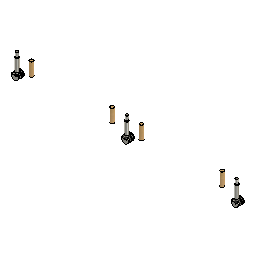
Minifix D15 Set (Autodesk Fusion 360 design; units mm, degrees)
description: Connecting Bolt
part number: L34
description: Dowel
part number: 8x30
description: Minifix CAM
part number: D15
description: Minifix Cap
part number: Minifix Cap D15
Autodesk Fusion 360 part; units mm, degrees
sketch "Main Area" plane through (0, 0, 0) normal (0, 0, 1) x (1, 0, 0)
  line L0 (300, 9) -> (-300, 9)
  line L1 (-300, 9) -> (-300, -9)
  line L2 (-300, -9) -> (300, -9)
  line L3 (300, -9) -> (300, 9)
  line L4 (300, 9) -> (-300, -9) construction
  line L5 (-300, 9) -> (300, -9) construction
  dimension "d3" = 600
  dimension "d4" = 18
  constraint horizontal L0
  constraint perpendicular L0 L1
  constraint parallel L0 L2
  constraint parallel L1 L3
  constraint coincident L4 origin
  constraint coincident L5 origin
  measures "d3" distance of L1.end L2.end
  measures "d4" distance of L0.end L1.end
sketch "Minfix Calc" plane through (0, 0, 0) normal (0, 0, 1) x (1, 0, 0)
  line L0 (0, 40) -> (0, -50)
  circle A0 centre (240, 1) radius 0.5
  line L1 (300, -9) -> (300, 9)
  line L2 (300, 9) -> (-300, 9)
  circle A1 centre (-240, 1) radius 0.5
  line L3 (-300, 9) -> (-300, -9)
  dimension "d7" = 1
  dimension "d8" = 60
  dimension "d9" = 8
  dimension "d18" = 1
  dimension "d19" = 8
  dimension "d20" = 60
  constraint vertical L0
  measures "d7" diameter of A0
  measures "d8" distance of A0.centre L1
  measures "d9" distance of A0.centre L2
  measures "d18" diameter of A1
  measures "d19" distance of L2 A1.centre
  measures "d20" distance of A1.centre L3
extrude "Extrude1" add sketch "Minfix Calc" along normal blind 10 contours A0 makes body 1
extrude "Extrude2" add sketch "Minfix Calc" along normal blind 10 separate body contours A1 makes body 2
sketch "Dowel Calc" plane through (0, 0, 0) normal (0, 0, 1) x (1, 0, 0)
  circle A0 centre (208, 1) radius 0.5
  circle A1 centre (240, 1) radius 0.5
  circle A2 centre (-208, 1) radius 0.5
  circle A3 centre (-240, 1) radius 0.5
  line L0 (-300, 9) -> (-300, -9)
  line L1 (300, -9) -> (300, 9)
  dimension "d23" = 1
  dimension "d25" = 1
  dimension "d55" = 92
  dimension "d56" = 92
  constraint horizontal A0.centre A1.centre
  constraint horizontal A2.centre A3.centre
  measures "d23" diameter of A0
  measures "d25" diameter of A2
  measures "d55" distance of A2.centre L0
  measures "d56" distance of A0.centre L1
extrude "Extrude3" add sketch "Dowel Calc" along normal blind 10 separate body contours A0 makes body 3
extrude "Extrude4" add sketch "Dowel Calc" along normal blind 10 separate body contours A2 makes body 4
pattern_linear "R-Pattern1" count 2 spacing 240 along (-1, 0, 0) of bodies 1 makes body 5
pattern_linear "R-Pattern3" count 2 spacing 240 along (-1, 0, 0) of bodies 3 makes body 6
pattern_linear "R-Pattern4" count 2 spacing 240 along (1, 0, 0) of bodies 4 makes body 7
sketch "Sketch6" plane through (0, 0, 0) normal (0, 0, 1) x (1, 0, 0)
  circle A0 centre (240, 1) radius 0.5
  circle A1 centre (240, 1) radius 2.5
  dimension "d57" = 5
  constraint concentric A0 A1
  measures "d57" diameter of A1
extrude "Extrude1'" add sketch "Sketch6" along normal blind 1.6 separate body contours A0 | A1 makes body 8 in component "Minifix Right"
sketch "Sketch1" plane through (0, 0, 1.6) normal (0, 0, 1) x (-1, 0, 0) in component "Minifix Right"
  circle A0 centre (-240, -1) radius 2.5
  circle A1 centre (-240, -1) radius 3
  dimension "d64" = 6
  constraint concentric A0 A1
  measures "d64" diameter of A1
extrude "Extrude2'" add sketch "Sketch1" along normal blind 9.4 contours A0 | A1 bodies 8 in component "Minifix Right"
chamfer "Chamfer1" distance 0.5 angle 45 1 edges at (242.797, 2.0848, 11) on bodies 8 in component "Minifix Right"
thread "Thread1" "ISO Metric profile 6.0 M6x1 6g" major diameter 5.884 minor diameter 4.7435 pitch 1 angle 60 resizes the face on face at (239.1875, -1.8879, 7.5333) on bodies 8 in component "Minifix Right"
sketch "Sketch2" plane through (0, 0, 0) normal (0, 0, -1) x (1, 0, 0) in component "Minifix Right"
  circle A0 centre (240, -1) radius 2.5
  circle A1 centre (240, -1) radius 2
  dimension "d68" = 4
  constraint concentric A0 A1
  measures "d68" diameter of A1
extrude "Extrude3'" add sketch "Sketch2" along normal blind 34 contours A1 bodies 8 in component "Minifix Right"
sketch "Sketch3" plane through (0, 0, -34) normal (0, 0, -1) x (1, 0, 0) in component "Minifix Right"
  circle A0 centre (240, -1) radius 2
  circle A1 centre (240, -1) radius 3.25
  line L0 (243.25, -1) -> (236.75, -1)
  dimension "d72" = 6.5
  constraint concentric A0 A1
  constraint horizontal L0
  constraint coincident A1 L0.start
  constraint coincident A1 L0.end
  constraint coincident A0.centre L0
  measures "d72" diameter of A1
revolve "Revolve1" add sketch "Sketch3" angle 180 about axis through (243.25, 1, -34) along (1, 0, 0) contours A0 A1 L0 picked at (237.1788, -1.1615) bodies 8 in component "Minifix Right"
sketch "Sketch4" plane through (0, 0, 0) normal (0, 0, -1) x (1, 0, 0) in component "Minifix Right"
  circle A0 centre (240, -1) radius 2
  circle A1 centre (240, -1) radius 2.5
  circle A2 centre (240, -1) radius 4
  dimension "d74" = 8
  constraint concentric A0 A2
  measures "d74" diameter of A2
ref_plane "WorkPlane1" through (240, 1, -26) normal (0, 0, -1) x (1, 0, 0) in component "Minifix Right"
extrude "Extrude4'" add sketch "Sketch4" along normal up to surface (26 mm away) contours A1 | A2 bodies 8 in component "Minifix Right"
sketch "Sketch5" plane through (0, 0, -34) normal (0, 0, -1) x (1, 0, 0) in component "Minifix Right"
  circle A0 centre (240, -1) radius 3.25
  line L0 (236.5, -0.5) -> (243.5, -0.5)
  line L1 (243.5, -0.5) -> (243.5, -1.5)
  line L2 (243.5, -1.5) -> (236.5, -1.5)
  line L3 (236.5, -1.5) -> (236.5, -0.5)
  line L4 (236.5, -0.5) -> (243.5, -1.5) construction
  line L5 (243.5, -0.5) -> (236.5, -1.5) construction
  line L6 (239.5, 2.5) -> (240.5, 2.5)
  line L7 (240.5, 2.5) -> (240.5, -4.5)
  line L8 (240.5, -4.5) -> (239.5, -4.5)
  line L9 (239.5, -4.5) -> (239.5, 2.5)
  line L10 (239.5, 2.5) -> (240.5, -4.5) construction
  line L11 (240.5, 2.5) -> (239.5, -4.5) construction
  point P0 (240, -1)
  point P1 (240, -1)
  dimension "d78" = 1
  dimension "d79" = 1
  dimension "d82" = 3.5
  dimension "d83" = 3.5
  constraint horizontal L0
  constraint perpendicular L0 L1
  constraint parallel L0 L2
  constraint parallel L1 L3
  constraint coincident L4 P1
  constraint coincident L5 P1
  constraint coincident P0 A0.centre
  constraint horizontal L6
  constraint perpendicular L6 L7
  constraint parallel L6 L8
  constraint parallel L7 L9
  constraint coincident L10 P1
  constraint coincident L11 P1
  constraint coincident P1 P0
  measures "d78" distance of L0.end L1.end
  measures "d79" distance of L7.end L8.end
  measures "d82" distance of L3 P1
  measures "d83" distance of P1 L8
extrude "Extrude5" cut sketch "Sketch5" against normal blind 1.5 draft -10 contours A0 L0 L2 L7 | A0 L0 L1 L2 | A0 L0 L7 L9 | A0 L6 L7 L9 | L0 L2 L7 L9 | A0 L7 L8 L9 | A0 L2 L7 L9 | A0 L0 L2 L9 | A0 L0 L2 L3 bodies 8 in component "Minifix Right"
sketch "Sketch6 (2)" plane through (0, 0, 0) normal (0, 0, 1) x (-1, 0, 0) in component "Minifix Right"
  circle A0 centre (-240, -1) radius 4
  circle A1 centre (-240, -1) radius 2.5
  circle A2 centre (-240, -1) radius 4
  dimension "d84" = 8
  constraint concentric A0 A2
  measures "d84" diameter of A2
extrude "Extrude6" add sketch "Sketch6 (2)" against normal blind 34 separate body contours A0 A2 | A1 makes body 9 in component "Minifix Right"
sketch "Sketch7" plane through (0, 0, 0) normal (0, 0, 1) x (-1, 0, 0) in component "Minifix Right"
  circle A0 centre (-240, -1) radius 4
  circle A1 centre (-240, -1) radius 2.5
  dimension "d87" = 5
  constraint concentric A0 A1
  measures "d87" diameter of A1
extrude "Extrude7" add sketch "Sketch7" along normal blind 13 contours A1 bodies 9 in component "Minifix Right"
pattern_linear "00000000-0000-0000-0000-000000000000" [suppressed]
sketch "Sketch7 (2)" plane through (0, 0, 0) normal (0, 0, 1) x (1, 0, 0)
  circle A0 centre (-240, 1) radius 0.5
  circle A1 centre (-240, 1) radius 2.5
  dimension "d94" = 5
  constraint concentric A0 A1
  measures "d94" diameter of A1
extrude "Extrude1''" add sketch "Sketch7 (2)" along normal blind 1.6 separate body contours A0 | A1 makes body 10 in component "Minifix left"
sketch "Sketch1 (2)" plane through (0, 0, 1.6) normal (0, 0, 1) x (-1, 0, 0) in component "Minifix left"
  circle A0 centre (240, -1) radius 2.5
  circle A1 centre (240, -1) radius 3
  dimension "d101" = 6
  constraint concentric A0 A1
  measures "d101" diameter of A1
extrude "Extrude2''" add sketch "Sketch1 (2)" along normal blind 9.4 contours A0 | A1 bodies 10 in component "Minifix left"
chamfer "Chamfer1'" distance 0.5 angle 45 1 edges at (-237.203, 2.0848, 11) on bodies 10 in component "Minifix left"
thread "Thread1'" "ISO Metric profile 6.0 M6x1 6g" major diameter 5.884 minor diameter 4.7435 pitch 1 angle 60 resizes the face on face at (-240.9555, -1.8438, 7.5333) on bodies 10 in component "Minifix left"
sketch "Sketch2 (2)" plane through (0, 0, 0) normal (0, 0, -1) x (1, 0, 0) in component "Minifix left"
  circle A0 centre (-240, -1) radius 2.5
  circle A1 centre (-240, -1) radius 2
  dimension "d105" = 4
  constraint concentric A0 A1
  measures "d105" diameter of A1
extrude "Extrude3''" add sketch "Sketch2 (2)" along normal blind 34 contours A1 bodies 10 in component "Minifix left"
sketch "Sketch5 (2)" plane through (0, 0, -34) normal (0, 0, -1) x (1, 0, 0) in component "Minifix left"
  circle A0 centre (-240, -1) radius 2
  line L0 (-236.75, -1) -> (-243.25, -1)
  arc A1 (-243.25, -1) -> (-236.75, -1) centre (-240, -1) ccw
  dimension "d110" = 6.5
  constraint concentric A0 A1
  constraint horizontal L0
  constraint coincident L0 A1.end
  constraint coincident L0 A1.start
  constraint coincident L0.start A1.end
  constraint coincident L0.end A1.start
  constraint coincident A0.centre L0
  measures "d110" diameter of A1
revolve "Revolve1'" add sketch "Sketch5 (2)" angle 180 about axis through (-236.75, 1, -34) along (1, 0, 0) contours A0 L0 A1 | A0 L0 picked at (-239.6702, -2.1926) bodies 10 in component "Minifix left"
sketch "Sketch6 (3)" plane through (0, 0, 0) normal (0, 0, -1) x (1, 0, 0) in component "Minifix left"
  circle A0 centre (-240, -1) radius 2
  circle A1 centre (-240, -1) radius 2.5
  circle A2 centre (-240, -1) radius 4
  dimension "d112" = 8
  constraint concentric A0 A2
  measures "d112" diameter of A2
extrude "Extrude4''" add sketch "Sketch6 (3)" along normal up to surface (26 mm away) contours A1 | A2 bodies 10 in component "Minifix left"
sketch "Sketch7 (3)" plane through (0, 0, -34) normal (0, 0, -1) x (1, 0, 0) in component "Minifix left"
  circle A0 centre (-240, -1) radius 3.25
  line L0 (-243.5, -0.5) -> (-236.5, -0.5)
  line L1 (-236.5, -0.5) -> (-236.5, -1.5)
  line L2 (-236.5, -1.5) -> (-243.5, -1.5)
  line L3 (-243.5, -1.5) -> (-243.5, -0.5)
  line L4 (-243.5, -0.5) -> (-236.5, -1.5) construction
  line L5 (-236.5, -0.5) -> (-243.5, -1.5) construction
  line L6 (-240.5, 2.5) -> (-239.5, 2.5)
  line L7 (-239.5, 2.5) -> (-239.5, -4.5)
  line L8 (-239.5, -4.5) -> (-240.5, -4.5)
  line L9 (-240.5, -4.5) -> (-240.5, 2.5)
  line L10 (-240.5, 2.5) -> (-239.5, -4.5) construction
  line L11 (-239.5, 2.5) -> (-240.5, -4.5) construction
  point P0 (-240, -1)
  point P1 (-240, -1)
  dimension "d115" = 1
  dimension "d116" = 1
  dimension "d119" = 3.5
  dimension "d120" = 3.5
  constraint horizontal L0
  constraint perpendicular L0 L1
  constraint parallel L0 L2
  constraint parallel L1 L3
  constraint coincident L4 P1
  constraint coincident L5 P1
  constraint coincident P0 A0.centre
  constraint horizontal L6
  constraint perpendicular L6 L7
  constraint parallel L6 L8
  constraint parallel L7 L9
  constraint coincident L10 P1
  constraint coincident L11 P1
  constraint coincident P1 P0
  measures "d115" distance of L0.end L1.end
  measures "d116" distance of L7.end L8.end
  measures "d119" distance of L3 P1
  measures "d120" distance of L8 P1
extrude "Extrude5'" cut sketch "Sketch7 (3)" against normal blind 1.5 draft -5 contours A0 L0 L2 L7 | A0 L0 L1 L2 | A0 L0 L7 L9 | A0 L6 L7 L9 | L0 L2 L7 L9 | A0 L7 L8 L9 | A0 L2 L7 L9 | A0 L0 L2 L9 | A0 L0 L2 L3 bodies 10 in component "Minifix left"
sketch "Sketch8" plane through (0, 0, 0) normal (0, 0, 1) x (-1, 0, 0) in component "Minifix left"
  circle A0 centre (240, -1) radius 4
  circle A1 centre (240, -1) radius 2.5
  circle A2 centre (240, -1) radius 4
  dimension "d121" = 8
  constraint concentric A0 A2
  measures "d121" diameter of A2
extrude "Extrude6'" add sketch "Sketch8" against normal blind 34 separate body contours A0 A2 | A1 makes body 11 in component "Minifix left"
sketch "Sketch9" plane through (0, 0, 0) normal (0, 0, 1) x (-1, 0, 0) in component "Minifix left"
  circle A0 centre (240, -1) radius 4
  circle A1 centre (240, -1) radius 2.5
  dimension "d124" = 5
  constraint concentric A0 A1
  measures "d124" diameter of A1
extrude "Extrude7'" add sketch "Sketch9" along normal blind 13 contours A1 bodies 11 in component "Minifix left"
sketch "Sketch8 (2)" plane through (0, 0, 0) normal (0, 0, 1) x (1, 0, 0)
  circle A0 centre (208, 1) radius 0.5
  circle A1 centre (208, 1) radius 4
  dimension "d132" = 8
  constraint concentric A0 A1
  measures "d132" diameter of A1
extrude "Extrude1'''" add sketch "Sketch8 (2)" along normal blind 10 and the other way blind 20 separate body contours A0 | A1 makes body 12 in component "Dowel Right"
chamfer "Chamfer1''" distance 0.5 angle 45 2 edges at (204.2707, 2.4465, -20) (204.2707, -0.4465, 10) on bodies 12 in component "Dowel Right"
extrude "Extrude2'''" add sketch "Sketch8 (2)" along normal blind -30 and the other way blind -12 separate body contours A0 | A1 makes body 13 in component "Dowel Right"
pattern_linear "00000000-0000-0000-0000-000000000000'" [suppressed]
sketch "Sketch9 (2)" plane through (0, 0, 10) normal (0, 0, 1) x (-1, 0, 0)
  circle A0 centre (208, -1) radius 0.5
  circle A1 centre (208, -1) radius 0.5
  circle A2 centre (208, -1) radius 4
  dimension "d150" = 8
  constraint concentric A1 A2
  measures "d150" diameter of A2
extrude "Extrude1''''" add sketch "Sketch9 (2)" along normal blind 10 and the other way blind 20 separate body contours A0 A1 | A2 makes body 14 in component "Dowel Left"
chamfer "Chamfer1'''" distance 0.5 angle 45 2 edges at (-204.2707, -0.4465, -10) (-204.2707, 2.4465, 20) on bodies 14 in component "Dowel Left"
extrude "Extrude2''''" add sketch "Sketch9 (2)" along normal blind 2 and the other way blind 40 separate body contours A0 A1 | A2 sketch seen with x (1, 0, 0) y (0, 1, 0) z (0, 0, 1) at (0, 0, 10) makes body 15 in component "Dowel Left"
pattern_linear "00000000-0000-0000-0000-000000000000''" [suppressed]
ref_plane "WorkPlane1" through (240, 1, -13) normal (0, 1, 0) x (0, 0, -1)
ref_plane "WorkPlane2" through (240, -3.5, -13) normal (0, 1, 0) x (0, 0, -1)
sketch "Sketch11" plane through (240, -3.5, -13) normal (0, 1, 0) x (1, 0, 0)
  line L0 (-0.5, 21) -> (0.5, 21) construction
  circle A0 centre (0, 21) radius 7.5
  point P0 (-0.5, 21)
  point P1 (0.5, 21)
  point P2 (0, 21)
  dimension "d170" = 15
  constraint coincident P0 L0.start
  constraint coincident P1 L0.end
  constraint midpoint L0 P2
  constraint coincident P2 A0.centre
  measures "d170" diameter of A0
extrude "Extrude1'''''" add sketch "Sketch11" along normal blind 12.5 separate body makes body 16 in component "Minifix CAM Right"
sketch "Sketch1 (3)" plane through (0, 9, 0) normal (0, 1, 0) x (-1, 0, 0) in component "Minifix CAM Right"
  circle A0 centre (-240, -34) radius 7.5
  circle A1 centre (-240, -34) radius 5.5 construction
  line L0 (-245.4486, -33.25) -> (-234.5514, -33.25)
  line L1 (-234.5514, -33.25) -> (-234.5514, -34.75)
  line L2 (-234.5514, -34.75) -> (-245.4486, -34.75)
  line L3 (-245.4486, -34.75) -> (-245.4486, -33.25)
  line L4 (-245.4486, -33.25) -> (-234.5514, -34.75) construction
  line L5 (-234.5514, -33.25) -> (-245.4486, -34.75) construction
  line L6 (-240.75, -39.4486) -> (-239.25, -39.4486)
  line L7 (-239.25, -39.4486) -> (-239.25, -28.5514)
  line L8 (-239.25, -28.5514) -> (-240.75, -28.5514)
  line L9 (-240.75, -28.5514) -> (-240.75, -39.4486)
  line L10 (-240.75, -39.4486) -> (-239.25, -28.5514) construction
  line L11 (-239.25, -39.4486) -> (-240.75, -28.5514) construction
  point P0 (-240, -34)
  point P1 (-240, -34)
  dimension "d174" = -2
  dimension "d175" = 1.5
  dimension "d176" = 1.5
  constraint horizontal L0
  constraint perpendicular L0 L1
  constraint parallel L0 L2
  constraint parallel L1 L3
  constraint coincident L4 P1
  constraint coincident L5 P1
  constraint coincident P0 A0.centre
  constraint horizontal L6
  constraint perpendicular L6 L7
  constraint parallel L6 L8
  constraint parallel L7 L9
  constraint coincident L10 P1
  constraint coincident L11 P1
  constraint coincident P1 P0
  constraint coincident A1 L6.end
  constraint coincident A1 L2.end
  measures "d175" distance of L0.end L1.end
  measures "d176" distance of L7.end L8.end
extrude "Extrude2'''''" cut sketch "Sketch1 (3)" against normal blind 2 draft -4 contours L0 L2 L3 L9 | L0 L7 L8 L9 | L0 L2 L7 L9 | L0 L1 L2 L7 | L2 L6 L7 L9 bodies 16 in component "Minifix CAM Right"
ref_plane "WorkPlane1" through (240, 3.5, -34) normal (0, 0, 1) x (0, 1, 0) in component "Minifix CAM Right"
sketch "Sketch2 (3)" plane through (240, 1.5, -34) normal (0, 0, 1) x (1, 0, 0) in component "Minifix CAM Right"
  circle A0 centre (0, -0.5) radius 2.25
  line L0 (7.5, 7.5) -> (-7.5, 7.5)
  line L1 (0, 1.75) -> (7.5, 1.75)
  line L2 (0, -2.75) -> (7.5, -2.75)
  line L3 (7.5, 7.5) -> (-7.5, 7.5)
  line L4 (7.5, -5) -> (-7.5, -5)
  line L5 (7.5, 7.5) -> (7.5, -5)
  line L6 (7.5, -5) -> (-7.5, -5)
  point P0 (0, -5)
  dimension "d181" = 4.5
  dimension "d182" = 8
  constraint horizontal L1
  constraint parallel L1 L2
  constraint tangent A0 L1
  constraint coincident A0 L1.start
  constraint coincident A0 L2.start
  constraint coincident L0.start L3.start
  constraint coincident L4.start L5.end
  constraint coincident L1.end L5
  constraint coincident L2.end L5
  constraint tangent A0 L2
  constraint midpoint L4 P0
  constraint vertical A0.centre P0
  measures "d181" diameter of A0
  measures "d182" distance of A0.centre L0
extrude "Extrude3'''" cut sketch "Sketch2 (3)" along normal mid plane 22 bodies 16 in component "Minifix CAM Right"
sketch "Sketch3 (2)" plane through (0, -3.5, 0) normal (0, -1, 0) x (1, 0, 0) in component "Minifix CAM Right"
  line L0 (245, -33) -> (235, -33)
  line L1 (235, -33) -> (235, -26.5)
  line L2 (235, -26.5) -> (245, -26.5)
  line L3 (245, -26.5) -> (245, -33)
  line L4 (245, -33) -> (235, -26.5) construction
  line L5 (235, -33) -> (245, -26.5) construction
  circle A0 centre (240, -34) radius 7.5
  circle A1 centre (240, -34) radius 7.5
  point P0 (240, -29.75)
  dimension "d186" = 10
  dimension "d274" = 6.5
  constraint horizontal L0
  constraint perpendicular L0 L1
  constraint parallel L0 L2
  constraint parallel L1 L3
  constraint coincident L4 P0
  constraint coincident L5 P0
  constraint tangent L2 A0
  constraint vertical P0 A0.centre
  measures "d186" distance of L1 L3
  measures "d274" distance of L0.end L1.end
extrude "Extrude4'''" cut sketch "Sketch3 (2)" against normal up to surface (6.75 mm away) contours L0 L1 L3 A0 A1 | L2 L3 A0 A1 | L1 L2 A0 A1 picked at (240, -30.8333) bodies 16 in component "Minifix CAM Right"
sketch "Sketch5 (3)" plane through (240, 1.5, -34) normal (0, 0, 1) x (1, 0, 0) in component "Minifix CAM Right"
  line L0 (5, -2.75) -> (5, -5)
  arc A0 (0, 1.75) -> (0, -2.75) centre (0, -0.5) ccw
  circle A1 centre (0, -0.5) radius 3.25
  line L1 (0, 2.75) -> (5, 2.75)
  line L2 (5, 2.75) -> (5, -3.75)
  line L3 (5, -3.75) -> (0, -3.75)
  line L4 (0, -3.75) -> (0, 2.75) construction
  line L5 (7.5, 1.75) -> (-5, 1.75)
  dimension "d191" = 6.5
  constraint concentric A0 A1
  constraint horizontal L1
  constraint vertical L2
  constraint horizontal L3
  constraint vertical L4
  constraint tangent A1 L1
  constraint tangent A1 L3
  constraint collinear L0 L2
  constraint coincident A0.centre L4
  measures "d191" diameter of A1
extrude "Extrude5''" cut sketch "Sketch5 (3)" along normal blind 7.5 and the other way blind 3 contours A1 L1 L2 L5 | A1 L5 | A1 L5 bodies 16 in component "Minifix CAM Right"
move_face "OffsetFaces1" offset -1 1 faces at (235.8849, 3.25, -31.4699) on bodies 16 in component "Minifix CAM Right"
fillet "Fillet1" radius 2 1 edges at (245, 3.75, -37) on bodies 16 in component "Minifix CAM Right"
fillet "Fillet1" radius 2 2 edges at (235, 0.375, -33) (245, -2.375, -33) on bodies 16 in component "Minifix CAM Right"
fillet "Fillet2" radius 1 4 edges at (237.0104, -0.2748, -37) (241.5, 4.25, -37) (244.4142, 4.25, -36.4142) (245, 4.25, -31.7049) on bodies 16 in component "Minifix CAM Right"
fillet "Fillet2" radius 1 3 edges at (238.5, 4.25, -33) (235.5858, 4.25, -32.4142) (235, 4.25, -29.7049) on bodies 16 in component "Minifix CAM Right"
ref_plane "WorkPlane2" through (240, 8, -34) normal (0, 1, 0) x (1, 0, 0) in component "Minifix CAM Right"
ref_plane "WorkPlane3" through (240, 5.25, -30.4688) normal (0, -1, 0) x (1, 0, 0) in component "Minifix CAM Right"
sketch "Sketch6 (4)" plane through (240, 8, -34) normal (0, 1, 0) x (1, 0, 0) in component "Minifix CAM Right"
  line L0 (0.6101, -0.6101) -> (5.3088, -0.6101)
  line L1 (0.6101, -5.3088) -> (0.6101, -0.6101)
  line L2 (-0.6101, -5.3088) -> (0.6101, -5.3088)
  line L3 (-0.6101, -0.6101) -> (-0.6101, -5.3088)
  line L4 (-5.3088, -0.6101) -> (-0.6101, -0.6101)
  line L5 (-0.6101, 0.6101) -> (-5.3088, 0.6101)
  line L6 (-5.3088, 0.6101) -> (-5.3088, -0.6101)
  line L7 (-0.6101, 5.3088) -> (-0.6101, 0.6101)
  line L8 (0.6101, 5.3088) -> (-0.6101, 5.3088)
  line L9 (0.6101, 0.6101) -> (0.6101, 5.3088)
  line L10 (5.3088, 0.6101) -> (0.6101, 0.6101)
  line L11 (5.3088, -0.6101) -> (5.3088, 0.6101)
  arc A0 (5, -5.5902) -> (0, 7.5) centre (0, 0) ccw
  spline S0 degree 3 poles (0, 7.5) (-0.2844, 7.5) (-0.5865, 7.4822) (-1.1404, 7.418) (-1.3922, 7.3725) (-1.7898, 7.2862) (-1.9627, 7.2396) (-2.1928, 7.1733) (-2.25, 7.1545) (-2.25, 7.1545) knots 0.341299 0.341299 0.341299 0.341299 0.426611 0.426611 0.511923 0.511923 0.59726 0.59726 0.682597 0.682597 0.682597 0.682597
  spline S1 degree 3 poles (-4, -6.3443) (-4.1326, -6.2607) (-4.2719, -6.1665) (-4.5277, -5.9812) (-4.6442, -5.8903) (-4.8117, -5.7539) (-4.8804, -5.6952) (-4.9747, -5.613) (-5, -5.5902) (-5, -5.5902) knots 0.161333 0.161333 0.161333 0.161333 0.208345 0.208345 0.255357 0.255357 0.293184 0.293184 0.331011 0.331011 0.331011 0.331011
  spline S2 degree 3 poles (5, -5.5902) (5, -5.5902) (4.9747, -5.613) (4.8804, -5.6952) (4.8117, -5.7539) (4.6442, -5.8903) (4.5277, -5.9812) (4.2719, -6.1665) (4.1326, -6.2607) (4, -6.3443) knots 0 0 0 0 0.037827 0.037827 0.075653 0.075653 0.122665 0.122665 0.169678 0.169678 0.169678 0.169678
  arc A1 (-4, -6.3443) -> (4, -6.3443) centre (0, 0) ccw
  arc A2 (-50.2768, -27.739) -> (-56.5684, 9.8605) centre (0, 0) ccw
  line L12 (-50.2768, -27.739) -> (-49.8166, 6.7466)
  spline S3 degree 3 poles (-49.8166, 6.7466) (-49.8164, 6.7433) (-49.8148, 6.716) (-49.8129, 6.668) (-49.8107, 6.6156) (-49.8082, 6.5341) (-49.8076, 6.4521) (-49.8068, 6.3498) (-49.8085, 6.2191) (-49.8151, 6.0836) (-49.8217, 5.9489) (-49.8338, 5.7996) (-49.849, 5.6667) knots 0.005365 0.005365 0.005365 0.005365 0.037827 0.037827 0.037827 0.075653 0.075653 0.075653 0.122665 0.122665 0.122665 0.169678 0.169678 0.169678 0.169678
  arc A3 (-49.9638, -4.5436) -> (-49.849, 5.6667) centre (0, 0) ccw
  spline S4 degree 3 poles (-49.9638, -4.5436) (-49.976, -4.4103) (-49.9848, -4.2608) (-49.9883, -4.126) (-49.9919, -3.9904) (-49.9907, -3.8597) (-49.9876, -3.7574) (-49.9851, -3.6755) (-49.9807, -3.5941) (-49.9774, -3.5417) (-49.9756, -3.5138) (-49.9742, -3.4929) (-49.9732, -3.4796) (-49.9727, -3.473) (-49.9723, -3.4683) (-49.9721, -3.4656) (-49.972, -3.4638) (-49.9719, -3.4629) (-49.9719, -3.4628) knots 0.161333 0.161333 0.161333 0.161333 0.208345 0.208345 0.208345 0.255357 0.255357 0.255357 0.293184 0.293184 0.293184 0.312097 0.312097 0.312097 0.321554 0.321554 0.321554 0.327733 0.327733 0.327733 0.327733
  arc A4 (-45.819, -9.949) -> (-45.6408, -10.7369) centre (0, 0) ccw
  line L13 (-1.6101, 6.3088) -> (-1.6101, 1.6101)
  line L14 (-1.6101, 1.6101) -> (-6.3088, 1.6101)
  line L15 (-6.3088, 1.6101) -> (-6.3088, -1.6101)
  line L16 (-6.3088, -1.6101) -> (-1.6101, -1.6101)
  line L17 (-1.6101, -1.6101) -> (-1.6101, -6.3088)
  line L18 (-1.6101, -6.3088) -> (1.6101, -6.3088)
  line L19 (1.6101, -6.3088) -> (1.6101, -1.6101)
  line L20 (1.6101, -1.6101) -> (6.3088, -1.6101)
  line L21 (6.3088, -1.6101) -> (6.3088, 1.6101)
  line L22 (6.3088, 1.6101) -> (1.6101, 1.6101)
  line L23 (1.6101, 1.6101) -> (1.6101, 6.3088)
  line L24 (1.6101, 6.3088) -> (-1.6101, 6.3088)
  arc A5 (5, -5.5902) -> (-5, -5.5902) centre (0, 0) ccw
  dimension "d209" = 1
  constraint concentric A0 A2
  constraint concentric A1 A3
  constraint tangent A3 S4
  constraint tangent S3 A3
  constraint concentric A4 A5
extrude "Extrude6''" cut sketch "Sketch6 (4)" against normal up to surface (2.75 mm away) contours A0 S0 S1 S2 A1 A5 bodies 16 in component "Minifix CAM Right"
sketch "Sketch7 (4)" plane through (0, 9, 0) normal (0, 1, 0) x (-1, 0, 0) in component "Minifix CAM Right"
  line L0 (-240.75, -28.5514) -> (-239.25, -28.5514)
  line L1 (-239.25, -28.5514) -> (-239.25, -33.25)
  line L2 (-239.25, -33.25) -> (-234.5514, -33.25)
  line L3 (-234.5514, -33.25) -> (-234.5514, -34.75)
  line L4 (-234.5514, -34.75) -> (-239.25, -34.75)
  line L5 (-239.25, -34.75) -> (-239.25, -39.4486)
  line L6 (-239.25, -39.4486) -> (-240.75, -39.4486)
  line L7 (-240.75, -39.4486) -> (-240.75, -34.75)
  line L8 (-240.75, -34.75) -> (-245.4486, -34.75)
  line L9 (-245.4486, -34.75) -> (-245.4486, -33.25)
  line L10 (-245.4486, -33.25) -> (-240.75, -33.25)
  line L11 (-240.75, -33.25) -> (-240.75, -28.5514)
  line L12 (-240.75, -28.5514) -> (-239.25, -28.5514)
  line L13 (-239.25, -28.5514) -> (-239.25, -33.25)
  line L14 (-239.25, -33.25) -> (-234.5514, -33.25)
  line L15 (-234.5514, -33.25) -> (-234.5514, -34.75)
  line L16 (-234.5514, -34.75) -> (-239.25, -34.75)
  line L17 (-239.25, -34.75) -> (-239.25, -39.4486)
  line L18 (-239.25, -39.4486) -> (-240.75, -39.4486)
  line L19 (-240.75, -39.4486) -> (-240.75, -34.75)
  line L20 (-240.75, -34.75) -> (-245.4486, -34.75)
  line L21 (-245.4486, -34.75) -> (-245.4486, -33.25)
  line L22 (-245.4486, -33.25) -> (-240.75, -33.25)
  line L23 (-240.75, -33.25) -> (-240.75, -28.5514)
  circle A0 centre (-240, -34) radius 7.5
  circle A1 centre (-240, -34) radius 7.5
  constraint concentric A0 A1
  constraint tangent A0 A1
extrude "Extrude7''" add sketch "Sketch7 (4)" along normal up to surface (-12.5 mm away) and the other way blind -0.1 separate body contours L0 L1 L2 L3 L4 L5 L6 L7 L8 L9 L10 L11 L12 L13 L14 L15 L16 L17 L18 L19 L20 L21 L22 L23 | A0 A1 makes body 17 in component "Minifix CAM Right"
pattern_linear "R-Pattern1'" [suppressed] in component "Minifix CAM Right"
sketch "Sketch12" plane through (240, -3.5, -13) normal (0, 1, 0) x (1, 0, 0)
  circle A0 centre (-480, 21) radius 7.5
  line L0 (-480.3688, 19.5) -> (-479.6312, 19.5)
  point P0 (-480.5, 21)
  point P1 (-480, 19.5)
  dimension "d220" = 15
  constraint horizontal A0.centre P0
  constraint midpoint L0 P1
  constraint vertical A0.centre P1
  measures "d220" diameter of A0
extrude "Extrude1''''''" add sketch "Sketch12" along normal blind 12.5 separate body makes body 18 in component "Minifix CAM Left"
sketch "Sketch1 (4)" plane through (0, 9, 0) normal (0, 1, 0) x (-1, 0, 0) in component "Minifix CAM Left"
  circle A0 centre (240, -34) radius 7.5
  circle A1 centre (240, -34) radius 7.5
  circle A2 centre (240, -34) radius 5.5 construction
  line L0 (234.5514, -33.25) -> (245.4486, -33.25)
  line L1 (245.4486, -33.25) -> (245.4486, -34.75)
  line L2 (245.4486, -34.75) -> (234.5514, -34.75)
  line L3 (234.5514, -34.75) -> (234.5514, -33.25)
  line L4 (234.5514, -33.25) -> (245.4486, -34.75) construction
  line L5 (245.4486, -33.25) -> (234.5514, -34.75) construction
  line L6 (239.25, -28.5514) -> (240.75, -28.5514)
  line L7 (240.75, -28.5514) -> (240.75, -39.4486)
  line L8 (240.75, -39.4486) -> (239.25, -39.4486)
  line L9 (239.25, -39.4486) -> (239.25, -28.5514)
  line L10 (239.25, -28.5514) -> (240.75, -39.4486) construction
  line L11 (240.75, -28.5514) -> (239.25, -39.4486) construction
  point P0 (240, -34)
  point P1 (240, -34)
  dimension "d223" = -2
  dimension "d224" = 1.5
  dimension "d225" = 1.5
  constraint horizontal L0
  constraint perpendicular L0 L1
  constraint parallel L0 L2
  constraint parallel L1 L3
  constraint coincident L4 P1
  constraint coincident L5 P1
  constraint coincident P1 P0
  constraint horizontal L6
  constraint perpendicular L6 L7
  constraint parallel L6 L8
  constraint parallel L7 L9
  constraint coincident L10 P1
  constraint coincident L11 P1
  constraint coincident A2 L8.end
  constraint coincident A2 L2.end
  measures "d224" distance of L0.end L1.end
  measures "d225" distance of L7.end L8.end
extrude "Extrude2''''''" cut sketch "Sketch1 (4)" against normal blind 2 draft -4 contours L0 L2 L3 L9 | L0 L6 L7 L9 | L0 L2 L7 L9 | L0 L1 L2 L7 | L2 L7 L8 L9 bodies 18 in component "Minifix CAM Left"
sketch "Sketch2 (4)" plane through (240, 1.5, -34) normal (0, 0, 1) x (1, 0, 0) in component "Minifix CAM Left"
  circle A0 centre (-480, -0.5) radius 2.25
  line L0 (-472.5, 7.5) -> (-487.5, 7.5)
  line L1 (-479.3899, 5.5) -> (-480.6101, 5.5)
  line L2 (-480, 1.75) -> (-472.5, 1.75)
  line L3 (-472.5, 1.75) -> (-472.5, -2.75)
  line L4 (-472.5, -2.75) -> (-480, -2.75)
  line L5 (-480, -2.75) -> (-480, 1.75)
  line L6 (-472.5, 7.5) -> (-472.5, -5)
  point P0 (-480, 5.5)
  dimension "d228" = 4.5
  dimension "d229" = 8
  constraint midpoint L1 P0
  constraint vertical A0.centre P0
  constraint horizontal L2
  constraint vertical L3
  constraint horizontal L4
  constraint vertical L5
  constraint coincident A0.centre L5
  constraint tangent A0 L2
  constraint tangent A0 L4
  constraint coincident L0.start L6.start
  constraint perpendicular L4 L6
  constraint collinear L3 L6
  measures "d228" diameter of A0
  measures "d229" distance of A0.centre L0
extrude "Extrude3''''" cut sketch "Sketch2 (4)" along normal through all and the other way through all bodies 18 in component "Minifix CAM Left"
sketch "Sketch3 (3)" plane through (0, -3.5, 0) normal (0, -1, 0) x (1, 0, 0) in component "Minifix CAM Left"
  line L0 (-235, -33) -> (-245, -33)
  line L1 (-245, -33) -> (-245, -26.5)
  line L2 (-245, -26.5) -> (-235, -26.5)
  line L3 (-235, -26.5) -> (-235, -33)
  line L4 (-235, -33) -> (-245, -26.5) construction
  line L5 (-245, -33) -> (-235, -26.5) construction
  circle A0 centre (-240, -34) radius 7.5
  circle A1 centre (-240, -34) radius 7.5
  point P0 (-240, -29.75)
  dimension "d232" = 10
  dimension "d275" = 6.5
  constraint horizontal L0
  constraint perpendicular L0 L1
  constraint parallel L0 L2
  constraint parallel L1 L3
  constraint coincident L4 P0
  constraint coincident L5 P0
  constraint vertical P0 A0.centre
  constraint tangent L2 A1
  measures "d232" distance of L1 L3
  measures "d275" distance of L0.end L1.end
extrude "Extrude4''''" cut sketch "Sketch3 (3)" against normal up to surface (6.75 mm away) contours L0 L1 L3 A0 A1 | L2 L3 A0 A1 | L1 L2 A0 A1 picked at (-240, -30.8333) bodies 18 in component "Minifix CAM Left"
sketch "Sketch4 (2)" plane through (0, 0, -33) normal (0, 0, 1) x (-1, 0, 0) in component "Minifix CAM Left"
  arc A0 (240, -3.25) -> (240, 1.25) centre (240, -1) ccw
  line L0 (240, -3.25) -> (245, -3.25)
  line L1 (245, -3.25) -> (245, 3.5)
  line L2 (245, 3.5) -> (235, 3.5)
  line L3 (235, 3.5) -> (235, 1.25)
  arc A1 (240, -3.25) -> (240, 1.25) centre (240, -1) ccw
  circle A2 centre (240, -1) radius 3.25
  line L4 (235, 2.25) -> (240, 2.25)
  line L5 (240, 2.25) -> (240, -4.25)
  line L6 (240, -4.25) -> (235, -4.25)
  line L7 (235, -4.25) -> (235, 2.25)
  line L8 (235, 2.25) -> (240, -4.25) construction
  line L9 (240, 2.25) -> (235, -4.25) construction
  line L10 (232.5, -3.25) -> (245, -3.25)
  line L11 (235, 3.5) -> (235, 1.25)
  line L12 (235, 1.25) -> (240, 1.25)
  point P0 (237.5, -1)
  dimension "d235" = 6.5
  constraint concentric A1 A2
  constraint horizontal L4
  constraint perpendicular L4 L5
  constraint parallel L4 L6
  constraint parallel L5 L7
  constraint coincident L8 P0
  constraint coincident L9 P0
  constraint coincident A0.centre L5
  constraint tangent A2 L6
  constraint tangent A2 L4
  measures "d235" diameter of A2
extrude "Extrude5'''" cut sketch "Sketch4 (2)" along normal blind 7.5 and the other way blind 3 contours A0 A1 L5 | A0 L0 A1 A2 L5 L10 | A2 L5 L10 L12 | L0 A2 L5 L10 | A2 L5 L10 | A2 L5 L12 | A2 L6 L7 L10 bodies 18 in component "Minifix CAM Left"
move_face "OffsetFaces1'" offset -1 1 faces at (-244.1151, 3.25, -31.4699) on bodies 18 in component "Minifix CAM Left"
fillet "Fillet1'" radius 2 3 edges at (-235, 3.75, -36) (-235, -2.375, -33) (-245, 0.375, -33) on bodies 18 in component "Minifix CAM Left"
fillet "Fillet2'" radius 1 7 edges at (-245, 4.25, -29.7049) (-244.4142, 4.25, -32.4142) (-241.5, 4.25, -33) (-242.9896, -0.2748, -36) (-238.5, 4.25, -36) (-235.5858, 4.25, -35.4142) (-235, 4.25, -31.2049) on bodies 18 in component "Minifix CAM Left"
ref_plane "WorkPlane1" through (-240, 8, -34) normal (0, 1, 0) x (1, 0, 0) in component "Minifix CAM Left"
ref_plane "WorkPlane2" through (-240, 5.25, -29.9688) normal (0, -1, 0) x (1, 0, 0) in component "Minifix CAM Left"
sketch "Sketch5 (4)" plane through (-240, 8, -34) normal (0, 1, 0) x (1, 0, 0) in component "Minifix CAM Left"
  arc A0 (5, -5.5902) -> (0, 7.5) centre (0, 0) ccw
  spline S0 degree 3 poles (0, 7.5) (-0.2844, 7.5) (-0.5865, 7.4822) (-1.1404, 7.418) (-1.3922, 7.3725) (-1.7898, 7.2862) (-1.9627, 7.2396) (-2.1928, 7.1733) (-2.25, 7.1545) (-2.25, 7.1545) knots 0.341299 0.341299 0.341299 0.341299 0.426611 0.426611 0.511923 0.511923 0.59726 0.59726 0.682597 0.682597 0.682597 0.682597
  arc A1 (-4, -6.3443) -> (4, -6.3443) centre (0, 0) ccw
  spline S1 degree 3 poles (-4, -6.3443) (-4.1256, -6.2651) (-4.2581, -6.1758) (-4.5032, -5.9995) (-4.6159, -5.9125) (-4.7897, -5.7723) (-4.8661, -5.7075) (-4.9714, -5.6161) (-5, -5.5902) (-5, -5.5902) knots 0.161333 0.161333 0.161333 0.161333 0.205875 0.205875 0.250417 0.250417 0.290759 0.290759 0.331101 0.331101 0.331101 0.331101
  spline S2 degree 3 poles (5, -5.5902) (5, -5.5902) (4.9747, -5.613) (4.8804, -5.6952) (4.8117, -5.7539) (4.6442, -5.8903) (4.5277, -5.9812) (4.2719, -6.1665) (4.1326, -6.2607) (4, -6.3443) knots 0 0 0 0 0.037827 0.037827 0.075653 0.075653 0.122665 0.122665 0.169678 0.169678 0.169678 0.169678
  arc A2 (35.2074, -13.7453) -> (35.5798, -12.7505) centre (0, 0) ccw construction
  line L0 (0.6101, 5.3088) -> (-0.6101, 5.3088)
  line L1 (-0.6101, 5.3088) -> (-0.6101, 0.6101)
  line L2 (-0.6101, 0.6101) -> (-5.3088, 0.6101)
  line L3 (-5.3088, 0.6101) -> (-5.3088, -0.6101)
  line L4 (-5.3088, -0.6101) -> (-0.6101, -0.6101)
  line L5 (-0.6101, -0.6101) -> (-0.6101, -5.3088)
  line L6 (-0.6101, -5.3088) -> (0.6101, -5.3088)
  line L7 (0.6101, -5.3088) -> (0.6101, -0.6101)
  line L8 (0.6101, -0.6101) -> (5.3088, -0.6101)
  line L9 (5.3088, -0.6101) -> (5.3088, 0.6101)
  line L10 (5.3088, 0.6101) -> (0.6101, 0.6101)
  line L11 (0.6101, 0.6101) -> (0.6101, 5.3088)
  line L12 (0.6101, 5.3088) -> (-0.6101, 5.3088)
  line L13 (-1.6101, 6.3088) -> (-1.6101, 1.6101)
  line L14 (-1.6101, 1.6101) -> (-6.3088, 1.6101)
  line L15 (-6.3088, 1.6101) -> (-6.3088, -1.6101)
  line L16 (-6.3088, -1.6101) -> (-1.6101, -1.6101)
  line L17 (-1.6101, -1.6101) -> (-1.6101, -6.3088)
  line L18 (-1.6101, -6.3088) -> (1.6101, -6.3088)
  line L19 (1.6101, -6.3088) -> (1.6101, -1.6101)
  line L20 (1.6101, -1.6101) -> (6.3088, -1.6101)
  line L21 (6.3088, -1.6101) -> (6.3088, 1.6101)
  line L22 (6.3088, 1.6101) -> (1.6101, 1.6101)
  line L23 (1.6101, 1.6101) -> (1.6101, 6.3088)
  line L24 (1.6101, 6.3088) -> (-1.6101, 6.3088)
  line L25 (11.0707, -9.5705) -> (18.0962, -3.2115)
  spline S3 degree 3 poles (18.0962, -3.2115) (18.0959, -3.2161) (18.0941, -3.2432) (18.0904, -3.2897) (18.0862, -3.342) (18.0789, -3.4232) (18.0696, -3.5047) (18.058, -3.6064) (18.0405, -3.7359) (18.0176, -3.8696) (17.9948, -4.0025) (17.9647, -4.1492) (17.9337, -4.2794) knots 0.006285 0.006285 0.006285 0.006285 0.037827 0.037827 0.037827 0.075653 0.075653 0.075653 0.122665 0.122665 0.122665 0.169678 0.169678 0.169678 0.169678 construction
  arc A3 (18.0793, -3.615) -> (17.9337, -4.2794) centre (0, 0) ccw construction
  spline S4 degree 3 poles (18.0793, -3.615) (18.1042, -3.4906) (18.1362, -3.3522) (18.1692, -3.2274) (18.2024, -3.102) (18.2386, -2.9816) (18.2695, -2.8862) (18.2974, -2.8003) (18.3274, -2.715) (18.3474, -2.66) (18.3581, -2.6308) (18.3663, -2.6088) (18.3716, -2.5947) (18.3743, -2.5877) (18.3762, -2.5827) (18.3773, -2.5798) (18.378, -2.578) (18.3784, -2.577) (18.3784, -2.5769) (18.3784, -2.5768) (18.3784, -2.5769) (18.3784, -2.5768) knots 0.161333 0.161333 0.161333 0.161333 0.205875 0.205875 0.205875 0.250417 0.250417 0.250417 0.290759 0.290759 0.290759 0.31093 0.31093 0.31093 0.321016 0.321016 0.321016 0.327264 0.327264 0.327264 0.327857 0.327857 0.327857 0.327857 construction
  arc A4 (31.9656, 20.3131) -> (33.3697, 17.9133) centre (0, 0) ccw construction
  line L26 (31.9656, 20.3131) -> (18.0962, -3.2115)
  arc A5 (5, -5.5902) -> (-5, -5.5902) centre (0, 0) ccw
  dimension "d249" = 1
  constraint concentric A2 A5
  constraint concentric A1 A3
  constraint concentric A0 A4
  constraint tangent A3 S4
  constraint tangent S3 A3
extrude "Extrude6'''" cut sketch "Sketch5 (4)" against normal up to surface (2.75 mm away) contours A0 S0 A1 S1 S2 A5 bodies 18 in component "Minifix CAM Left"
sketch "Sketch6 (5)" plane through (0, 9, 0) normal (0, 1, 0) x (-1, 0, 0) in component "Minifix CAM Left"
  line L0 (240.75, -34.75) -> (240.75, -39.4486)
  line L1 (240.75, -39.4486) -> (239.25, -39.4486)
  line L2 (239.25, -39.4486) -> (239.25, -34.75)
  line L3 (239.25, -34.75) -> (234.5514, -34.75)
  line L4 (234.5514, -34.75) -> (234.5514, -33.25)
  line L5 (234.5514, -33.25) -> (239.25, -33.25)
  line L6 (239.25, -33.25) -> (239.25, -28.5514)
  line L7 (239.25, -28.5514) -> (240.75, -28.5514)
  line L8 (240.75, -28.5514) -> (240.75, -33.25)
  line L9 (240.75, -33.25) -> (245.4486, -33.25)
  line L10 (245.4486, -33.25) -> (245.4486, -34.75)
  line L11 (245.4486, -34.75) -> (240.75, -34.75)
  circle A0 centre (240, -34) radius 7.5
  circle A1 centre (240, -34) radius 7.5
extrude "Extrude7'''" add sketch "Sketch6 (5)" against normal blind 12.5 separate body contours L0 L1 L2 L3 L4 L5 L6 L7 L8 L9 L10 L11 | A0 A1 makes body 19 in component "Minifix CAM Left"
sketch "Sketch13" plane through (0, 9, 0) normal (0, 1, 0) x (-1, 0, 0)
  line L0 (-240.75, -28.5514) -> (-239.25, -28.5514)
  line L1 (-239.25, -28.5514) -> (-239.25, -33.25)
  line L2 (-239.25, -33.25) -> (-234.5514, -33.25)
  line L3 (-234.5514, -33.25) -> (-234.5514, -34.75)
  line L4 (-234.5514, -34.75) -> (-239.25, -34.75)
  line L5 (-239.25, -34.75) -> (-239.25, -39.4486)
  line L6 (-239.25, -39.4486) -> (-240.75, -39.4486)
  line L7 (-240.75, -39.4486) -> (-240.75, -34.75)
  line L8 (-240.75, -34.75) -> (-245.4486, -34.75)
  line L9 (-245.4486, -34.75) -> (-245.4486, -33.25)
  line L10 (-245.4486, -33.25) -> (-240.75, -33.25)
  line L11 (-240.75, -33.25) -> (-240.75, -28.5514)
  circle A0 centre (-240, -34) radius 7.5
  circle A1 centre (-240, -34) radius 7.5
  line L12 (-240.75, -28.5514) -> (-239.25, -28.5514)
  line L13 (-239.25, -28.5514) -> (-239.25, -33.25)
  line L14 (-239.25, -33.25) -> (-234.5514, -33.25)
  line L15 (-234.5514, -33.25) -> (-234.5514, -34.75)
  line L16 (-234.5514, -34.75) -> (-239.25, -34.75)
  line L17 (-239.25, -34.75) -> (-239.25, -39.4486)
  line L18 (-239.25, -39.4486) -> (-240.75, -39.4486)
  line L19 (-240.75, -39.4486) -> (-240.75, -34.75)
  line L20 (-240.75, -34.75) -> (-245.4486, -34.75)
  line L21 (-245.4486, -34.75) -> (-245.4486, -33.25)
  line L22 (-245.4486, -33.25) -> (-240.75, -33.25)
  line L23 (-240.75, -33.25) -> (-240.75, -28.5514)
  circle A2 centre (-240, -34) radius 7.5
extrude "Extrude1'''''''" add sketch "Sketch13" along normal blind 1.5 separate body contours L0 L1 L2 L3 L4 L5 L6 L7 L8 L9 L10 L11 L12 L13 L14 L15 L16 L17 L18 L19 L20 L21 L22 L23 | A0 A1 A2 makes body 20 in component "Cap"
fillet "Fillet1''" radius 1 1 edges at (246.9925, 10.5, -36.7121) on bodies 20 in component "Cap"
pattern_linear "00000000-0000-0000-0000-000000000000'''" [suppressed]
pattern_linear "00000000-0000-0000-0000-000000000000''''" [suppressed]
component "Minifix Right" placed x (1, 0, 0) y (0, 1, 0) z (0, 0, 1) at (0, 0, 0)
component "Minifix left" placed x (1, 0, 0) y (0, 1, 0) z (0, 0, 1) at (0, 0, 0)
component "Minifix Right" placed x (1, 0, 0) y (0, 1, 0) z (0, 0, 1) at (-240, 0, 0)
component "Dowel Right" placed x (1, 0, 0) y (0, 1, 0) z (0, 0, 1) at (0, 0, 0)
component "Dowel Left" placed x (1, 0, 0) y (0, 1, 0) z (0, 0, 1) at (0, 0, -10)
component "Dowel Right" placed x (1, 0, 0) y (0, 1, 0) z (0, 0, 1) at (-240, 0, 0)
component "Minifix CAM Right" placed x (1, 0, 0) y (0, 1, 0) z (0, 0, 1) at (0, 0, 0)
component "Dowel Left" placed x (1, 0, 0) y (0, 1, 0) z (0, 0, 1) at (240, 0, -10)
component "Minifix CAM Left" placed x (1, 0, 0) y (0, 1, 0) z (0, 0, 1) at (0, 0, 0)
component "Cap" placed x (1, 0, 0) y (0, 1, 0) z (0, 0, 1) at (0, 0, 0)
component "Cap" placed x (1, 0, 0) y (0, 1, 0) z (0, 0, 1) at (-480, 0, 0)
component "Cap" placed x (1, 0, 0) y (0, 1, 0) z (0, 0, 1) at (-240, 0, 0)
component "Minifix CAM Right" placed x (1, 0, 0) y (0, 1, 0) z (0, 0, 1) at (-240, 0, 0)
hidden bodies 1 2 3 4 5 6 7 9 11 13 15 19
equation "ContactPatchLength = 600 mm"
equation "ContactPatchWidth = 18 mm"
equation "d3 = ContactPatchLength"
equation "d4 = ContactPatchWidth"
equation "Y_Coord = ( if(ContactPatchWidth < 13 mm; 6; if(ContactPatchWidth >= 13 mm and ContactPatchWidth < 16 mm; 6.5; if(ContactPatchWidth >= 16 mm and ContactPatchWidth < 19 mm; 8; if(ContactPatchWidth >= 19 mm and ContactPatchWidth < 23 mm; 9.5; if(ContactPatchWidth >= 23 mm and ContactPatchWidth < 29 mm; 11.5; if(ContactPatchWidth >= 29 mm; 14.5; 9.5)))))) ) * 1 mm"
equation "d8 = DistFromSide1"
equation "d9 = Y_Coord"
equation "DistFromSide1 = 60 mm" comment "Distance from the Edge"
equation "DistFromSide2 = 60 mm" comment "Distance from the Edge"
equation "d19 = Y_Coord"
equation "d20 = DistFromSide2"
equation "NumberOfComponents = if(ContactPatchLength >= 600 mm; 2; 1)"
equation "DistToNextComponent = ( ContactPatchLength / 2 ) - DistFromSide1"
equation "d33 = NumberOfComponents"
equation "d35 = DistToNextComponent"
equation "d47 = NumberOfComponents"
equation "d49 = -DistToNextComponent"
equation "d51 = NumberOfComponents"
equation "d53 = DistToNextComponent"
equation "d55 = DistFromSide2 + 32 mm"
equation "d56 = DistFromSide1 + 32 mm"
equation "BoltLength = 34 mm" comment "Connecting Bolt Length 34 mm"
equation "d70 = BoltLength"
equation "d83 = d82"
equation "d85 = -BoltLength"
equation "d90 = NumberOfComponents"
equation "d92 = -DistToNextComponent"
equation "d106 = BoltLength"
equation "d122 = -BoltLength"
equation "DowelDia = 8 mm" comment "Dowel diameter 8 mm"
equation "d132 = DowelDia"
equation "d146 = NumberOfComponents"
equation "d148 = -DistToNextComponent"
equation "d150 = DowelDia"
equation "d164 = NumberOfComponents"
equation "d166 = DistToNextComponent"
equation "DrillingDepth = ( if(ContactPatchWidth < 13 mm; 9.5; if(ContactPatchWidth >= 13 mm and ContactPatchWidth < 16 mm; 11; if(ContactPatchWidth >= 16 mm and ContactPatchWidth < 19 mm; 12.5; if(ContactPatchWidth >= 19 mm and ContactPatchWidth < 23 mm; 14; if(ContactPatchWidth >= 23 mm and ContactPatchWidth < 29 mm; 16.5; if(ContactPatchWidth >= 29 mm; 19.5; 19.5)))))) ) * 1 mm" comment "Board thickness up to 19 mm"
equation "d172 = DrillingDepth"
equation "PinPosition = Y_Coord" comment "Board thickness up to 16 mm"
equation "d182 = PinPosition"
equation "d192 = ( 15 / 2 ) * 1 mm"
equation "d216 = NumberOfComponents"
equation "d218 = -DistToNextComponent"
equation "d221 = DrillingDepth"
equation "d229 = PinPosition"
equation "d236 = ( 15 / 2 ) * 1 mm"
equation "d252 = -DrillingDepth"
equation "d266 = NumberOfComponents"
equation "d268 = -DistToNextComponent"
equation "d270 = NumberOfComponents"
equation "d272 = -DistToNextComponent"
named bodies: "Minfix Right", "Minifix Left", "Dowel Right", "Dowel Left", "Connecting Bolt", "Bolt Hole", "Dowel", "Dowel Hole", "CAM", "CAM Hole", "CAM (1)", "Minfix Right (1)", "Dowel Right (1)", "Dowel Left (1)"
